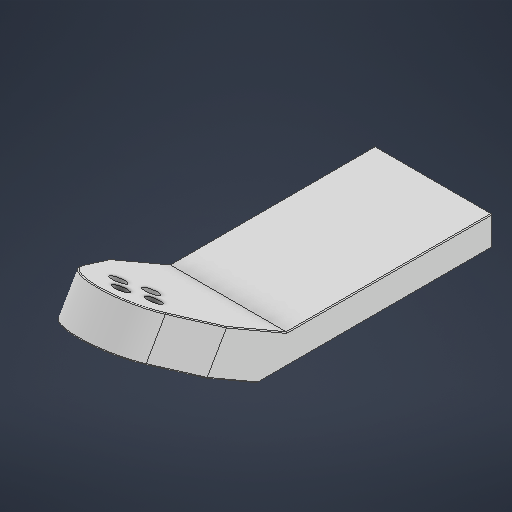
# Autodesk Inventor part: rearTorso60Deg
Saved by Autodesk Inventor 2026 (Build 300175000, 175)
## iProperties
Created: 2025-05-30
Part Number: rearTorso60Deg
Material: Generic
Document SubType Name: Modeling
Designer: Elizabeth
Density: 1 g/cm^3
Appearance: Default
Author: Elizabeth
Autodesk Inventor part; units mm, degrees
ref_plane "YZ Plane" through (0, 0, 0) normal (1, 0, 0) x (0, 1, 0)
ref_plane "XZ Plane" through (0, 0, 0) normal (0, 1, 0) x (-1, 0, 0)
ref_plane "XY Plane" through (0, 0, 0) normal (0, 0, 1) x (1, 0, 0)
sketch "Sketch1" plane through (0, 0, 0) normal (1, 0, 0) x (0, 1, 0)
  line L0 (0, -80) -> (0, 0)
  line L1 (0, -80) -> (10, -80)
  line L2 (10, -80) -> (10, 17.3205)
  line L3 (10, -10) -> (35.6301, 34.3927)
  line L4 (0, 0) -> (10, 17.3205)
  line L5 (10, 17.3205) -> (23.8, 41.2228)
  line L6 (23.8, 41.2228) -> (35.6301, 34.3927)
  dimension "d2" = 10
  dimension "d6" = 27.6
  constraints: 14 end point, 2 perpendicular, 1 parallel, 1 point on line
  measures "d2" distance of L0.start L1.end
  measures "d6" distance of L2.end L5.end
extrude "Extrusion1" add sketch "Sketch1" against normal blind 40
sketch "Sketch2" plane through (-40, 23.8, 41.2228) normal (0, -0.8660254, 0.5) x (1, 0, 0)
  line L0 (40, 0) -> (0, 0)
  line L1 (0, -27.6) -> (40, -27.6)
  line L2 (0, -27.6) -> (0, 0)
  line L3 (40, 0) -> (40, -27.6)
  circle A0 centre (20, -15) radius 15
  circle A1 centre (20, -15) radius 8.5
  line L4 (0, -27.6) -> (0, 0)
  line L5 (0, -27.6) -> (5.7669, -10.265)
  line L6 (40, -27.6) -> (34.2331, -10.265)
  circle A2 centre (20, -15) radius 6
  circle A3 centre (20, -9) radius 1.2
  circle A4 centre (26, -15) radius 1.2
  circle A5 centre (20, -21) radius 1.2
  circle A6 centre (14, -15) radius 1.2
  line L7 (40, 0) -> (0, 0) projected
  line L8 (0, 0) -> (-36.8093, 14.5426)
  point P0 (40, -47.6)
  point P1 (20, 0)
  dimension "d9" = 30
  dimension "d10" = 17
  dimension "d11" = 12
  dimension "d12" = 2.4
  dimension "d13" = 2.4
  dimension "d14" = 2.4
  dimension "d15" = 2.4
  constraints: 16 end point, 7 centre point, 6 point on circle, 2 coincident, 2 tangent, 1 parallel, 1 perpendicular
  measures "d9" diameter of A0
  measures "d10" diameter of A1
  measures "d11" diameter of A2
  measures "d12" diameter of A3
  measures "d13" diameter of A4
  measures "d14" diameter of A5
  measures "d15" diameter of A6
extrude "Extrusion2" cut sketch "Sketch2" against normal up to surface (13.6603 mm away) contours L3 L6 A0 L0 | A0 L5 L2 L0 | A2 A4 | A2 A4 | A3 A2 | A2 A3 | A5 A2 | A2 A5 | A6 A2 | A2 A6
sketch "Sketch3" plane through (-40, 10, -10) normal (0, 0.8660254, -0.5) x (1, 0, 0)
  circle A0 centre (14, -36.2603) radius 1.2 projected
  circle A1 centre (14, -36.2603) radius 2.5
  circle A2 centre (20, -30.2603) radius 1.2 projected
  circle A3 centre (20, -30.2603) radius 2.5
  circle A4 centre (26, -36.2603) radius 1.2 projected
  circle A5 centre (26, -36.2603) radius 2.5
  circle A6 centre (20, -42.2603) radius 1.2 projected
  circle A7 centre (20, -42.2603) radius 2.5
  point P0 (40, -3.6603)
  dimension "d18" = 5
  dimension "d19" = 5
  dimension "d20" = 5
  constraints: 4 centre point, 4 coincident
  measures "d18" diameter of A1
  measures "d19" diameter of A3
  measures "d20" diameter of A7
extrude "Extrusion3" cut sketch "Sketch3" against normal blind 2 contours A0 | A1 | A2 | A3 | A4 | A5 | A6 | A7
fillet "Fillet1" radius 0.3 19 edges at (-2.8835, 26.1639, 17.9967) (-37.1165, 26.1639, 17.9967) (-20, 35.6301, 34.3927) (0, 15.9151, 0.2452) (0, 5, 8.6603) (-20, 23.8, 41.2228) (-37.1165, 14.3338, 24.8268) (-2.8835, 14.3338, 24.8268) (0, 10, -45) (-20, 0, 0) (0, 0, -40) (-40, 5, 8.6603) (-40, 15.9151, 0.2452) (-40, 10, -45) (-40, 0, -40) (-40, 5, -80) (-20, 10, -80) (-20, 0, -80) (0, 5, -80)
extrude "Extrusion4" cut sketch "Sketch2" against normal blind 2.5 contours A1 | A2 A4 | A2 A4 | A4 A2 A5 A6 A3 | A3 A2 | A2 A3 | A5 A2 | A2 A5 | A6 A2 | A2 A6
body "Solid1"
